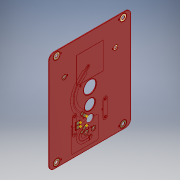
# Autodesk Inventor part: +XPanel_PCB
Saved by Autodesk Inventor 2018 (Build 220112000, 112)
## iProperties
Created: 2018-07-05
Part Number: +XPanel_PCB
Material: Epoxy Resin
Document SubType Name: Modeling
Designer: Bradley
Density: 1.14 g/cm^3
Appearance: Smooth - Red
Mass: 8.24144 g
Surface Area: 149.532 cm^2
Volume: 7.22933 cm^3
Author: Bradley
Autodesk Inventor part; units mm, degrees
(part 1 of 2)
ref_plane "YZ Plane" through (0, 0, 0) normal (1, 0, 0) x (0, 1, 0)
ref_plane "XZ Plane" through (0, 0, 0) normal (0, 1, 0) x (-1, 0, 0)
ref_plane "XY Plane" through (0, 0, 0) normal (0, 0, 1) x (1, 0, 0)
sketch "Sketch1" plane through (0, 0, 0) normal (1, 0, 0) x (0, 1, 0)
  line L0 (-35, -49.5) -> (35, -49.5)
  line L1 (40, -44.5) -> (40, 44.5)
  line L2 (35, 49.5) -> (-35, 49.5)
  line L3 (-40, 44.5) -> (-40, -44.5)
  line L4 (-40, -49.5) -> (40, 49.5) construction
  line L5 (40, -49.5) -> (-40, 49.5) construction
  arc A0 (-35, 49.5) -> (-40, 44.5) centre (-35, 44.5) ccw
  arc A1 (40, 44.5) -> (35, 49.5) centre (35, 44.5) ccw
  arc A2 (35, -49.5) -> (40, -44.5) centre (35, -44.5) ccw
  arc A3 (-40, -44.5) -> (-35, -49.5) centre (-35, -44.5) ccw
  point P0 (0, 0)
  dimension "d0" = 80
  dimension "d1" = 99
  dimension "d2" = 5
  constraints: 12 end point, 8 point on circle, 8 point on line, 8 tangent, 4 centre point, 3 equal radius, 2 midpoint, 2 parallel, 1 horizontal, 1 perpendicular
  measures "d0" distance of L4.end L5.end
  measures "d1" distance of L5.end L4.start
  measures "d2" radius of A0
extrude "Extrusion1" add sketch "Sketch1" along normal mid plane 0.5
sketch "Sketch2" plane through (0.25, 0, 0) normal (1, 0, 0) x (0, 0, -1)
  line L0 (45, -32.5) -> (-45, -32.5) construction
  line L1 (-45, -32.5) -> (-45, 32.5) construction
  line L2 (-45, 32.5) -> (45, 32.5) construction
  line L3 (45, 32.5) -> (45, -32.5) construction
  line L4 (45, -32.5) -> (-45, 32.5) construction
  line L5 (-45, -32.5) -> (45, 32.5) construction
  point P0 (0, 0)
  dimension "d5" = 90
  dimension "d6" = 65
  constraints: 12 end point, 4 coincident, 2 midpoint, 2 parallel, 1 horizontal, 1 perpendicular
  measures "d5" distance of L1.end L2.end
  measures "d6" distance of L0.end L1.end
hole "Hole1" at (0.25, -32.5, 45) at (0.25, 32.5, 45) at (0.25, 32.5, -45) at (0.25, -32.5, -45) direction (-1, 0, 0) diameter 3.3 end through all
sketch "Sketch3" plane through (0.25, 0, 0) normal (1, 0, 0) x (0, 0, -1)
  circle A0 centre (-2.5, 0) radius 6
  circle A1 centre (12.35, 0) radius 5
  circle A2 centre (-21, -1.75) radius 0.475
  circle A3 centre (24, 0) radius 3.5
  circle A4 centre (38.6, 1) radius 0.4572
  circle A5 centre (38.6, -1) radius 0.4572
  line L0 (38.6, -1) -> (38.6, 1) construction
  line L1 (38.6, 1) -> (38.6, 5.5714) construction
  line L2 (34.1, -3.5714) -> (34.1, 3.5714) construction
  line L3 (-23.3841, -25.0749) -> (-23.3841, 25.0749) construction
  line L4 (-2.5, 0) -> (-37.3972, 41.9) construction
  line L5 (-40, 41.9) -> (-5.1028, 0) construction
  line L6 (15, -15) -> (30, -15) construction
  line L7 (30, -15) -> (30, 15) construction
  line L8 (30, 15) -> (15, 15) construction
  line L9 (15, 15) -> (15, -15) construction
  circle A6 centre (15, -15) radius 0.5
  circle A7 centre (30, -15) radius 0.5
  circle A8 centre (30, 15) radius 0.5
  circle A9 centre (15, 15) radius 0.5
  circle A10 centre (0, 0) radius 39 construction
  circle A11 centre (0, 0) radius 34.2865 construction
  point P0 (38.6, 0)
  point P1 (34.1, 0)
  point P2 (30, 0)
  dimension "d53" = 78
  dimension "d14" = 14.85
  dimension "d15" = 12
  dimension "d16" = 10
  dimension "d19" = 2.5
  dimension "d20" = 21
  dimension "d21" = 1.75
  dimension "d22" = 0.95
  dimension "d23" = 7
  dimension "d24" = 26.5
  dimension "d25" = 0.9144
  dimension "d26" = 2
  dimension "d27" = 38.6
  dimension "d28" = 4.5714
  dimension "d34" = 4.5
  dimension "d46" = 2
  dimension "d47" = 41.9
  dimension "d49" = 15
  dimension "d50" = 1
  dimension "d51" = 30
  dimension "d52" = 15
  dimension "d54" = 40
  dimension "d55" = 2
  constraints: 20 end point, 11 centre point, 8 horizontal alignment, 6 coincident, 4 equal radius, 4 vertical, 3 midpoint, 3 parallel, 3 point on circle, 1 horizontal, 1 perpendicular, 1 point on line, 3 other
  measures "d14" distance of A1.centre point (-2.5, 0)
  measures "d15" diameter of A0
  measures "d16" diameter of A1
  measures "d19" distance of point (0, 0) point (-2.5, 0)
  measures "d20" horizontal distance of point (0, 0) A2.centre
  measures "d21" vertical distance of point (0, 0) A2.centre
  measures "d22" diameter of A2
  measures "d23" diameter of A3
  measures "d24" distance of A3.centre point (-2.5, 0)
  measures "d25" diameter of A4
  measures "d26" distance of L0.start L0.end
  measures "d27" distance from line of point (0, 0) L0
  measures "d28" distance of L0.end L1.end
  measures "d34" distance between parallel lines of L0 L2
  measures "d46" distance between parallel lines of L4 L5
  measures "d47" vertical distance of L4.start L4.end
  measures "d49" distance of L8.end L7.end
  measures "d50" diameter of A6
  measures "d51" distance of L6.end L7.end
  measures "d52" distance from line of point (0, 0) L9
  measures "d54" horizontal distance of point (0, 0) L5.start
  measures "d55" vertical distance of L2.end L1.end
extrude "Extrusion2" cut sketch "Sketch3" against normal through all
sketch "Sketch4" plane through (0.25, 0, 0) normal (1, 0, 0) x (0, 0, -1)
  point P0 (0, 0)
  point P1 (34.1, -3.5714)
  point P2 (34.1, 3.5714)
  point P3 (-23.3841, -25.0749)
  point P4 (-23.3841, 25.0749)
hole "Hole2" at (0.25, -3.5714, -34.1) at (0.25, 3.5714, -34.1) at (0.25, -25.0749, 23.3841) at (0.25, 25.0749, 23.3841) direction (-1, 0, 0) diameter 2.2 end through all clearance for "Flat Head Machine Screw" size "M2" standard "Ansi Metric M Profile"
sketch "Sketch5" plane through (0.25, 0, 0) normal (1, 0, 0) x (0, 0, -1)
  circle A0 centre (-23.3841, -25.0749) radius 1.1 projected
  circle A1 centre (34.1, -3.5714) radius 1.1 projected
  circle A2 centre (34.1, 3.5714) radius 1.1 projected
  circle A3 centre (-23.3841, 25.0749) radius 1.1 projected
  circle A4 centre (12.35, 0) radius 5 projected
  circle A5 centre (15, 15) radius 0.5 projected
  circle A6 centre (30, -15) radius 0.5 projected
  circle A7 centre (-21, -1.75) radius 0.475 projected
  circle A8 centre (38.6, 1) radius 0.4572 projected
  circle A9 centre (38.6, -1) radius 0.4572 projected
  circle A10 centre (15, -15) radius 0.5 projected
  circle A11 centre (30, 15) radius 0.5 projected
  circle A12 centre (24, 0) radius 3.5 projected
  circle A13 centre (-2.5, 0) radius 6 projected
  circle A14 centre (45, 32.5) radius 1.65 projected
  circle A15 centre (-45, -32.5) radius 1.65 projected
  circle A16 centre (-45, 32.5) radius 1.65 projected
  circle A17 centre (45, -32.5) radius 1.65 projected
  line L0 (-44.5, -40) -> (44.5, -40) projected
  arc A18 (44.5, -40) -> (49.5, -35) centre (44.5, -35) ccw projected
  line L1 (49.5, -35) -> (49.5, 35) projected
  arc A19 (49.5, 35) -> (44.5, 40) centre (44.5, 35) ccw projected
  line L2 (44.5, 40) -> (-44.5, 40) projected
  arc A20 (-44.5, 40) -> (-49.5, 35) centre (-44.5, 35) ccw projected
  line L3 (-49.5, 35) -> (-49.5, -35) projected
  arc A21 (-49.5, -35) -> (-44.5, -40) centre (-44.5, -35) ccw projected
  circle A22 centre (-45, -32.5) radius 1.65 projected
  circle A23 centre (-45, -32.5) radius 3
  circle A24 centre (-23.3841, -25.0749) radius 1.1 projected
  circle A25 centre (-23.3841, -25.0749) radius 2
  circle A26 centre (-45, 32.5) radius 1.65 projected
  circle A27 centre (-45, 32.5) radius 3
  circle A28 centre (-23.3841, 25.0749) radius 1.1 projected
  circle A29 centre (-23.3841, 25.0749) radius 2
  circle A30 centre (34.1, 3.5714) radius 1.1 projected
  circle A31 centre (34.1, 3.5714) radius 2
  circle A32 centre (34.1, -3.5714) radius 1.1 projected
  circle A33 centre (34.1, -3.5714) radius 2
  circle A34 centre (45, -32.5) radius 3
  circle A35 centre (45, 32.5) radius 1.65 projected
  circle A36 centre (45, 32.5) radius 3
  circle A37 centre (38.6, -1) radius 0.85
  circle A38 centre (38.6, 1) radius 0.4572 projected
  circle A39 centre (38.6, 1) radius 0.85
  circle A40 centre (30, 15) radius 0.9
  circle A41 centre (15, 15) radius 0.5 projected
  circle A42 centre (15, 15) radius 0.9
  circle A43 centre (30, -15) radius 0.5 projected
  circle A44 centre (30, -15) radius 0.9
  circle A45 centre (15, -15) radius 0.5 projected
  circle A46 centre (15, -15) radius 0.9
  line L4 (22.9, -12) -> (25.1, -12) construction
  line L5 (25.1, -12) -> (25.1, -10) construction
  line L6 (25.1, -10) -> (22.9, -10) construction
  line L7 (22.9, -10) -> (22.9, -12) construction
  line L8 (22.75, -9) -> (25.25, -9) construction
  line L9 (25.25, -9) -> (25.25, -5.5) construction
  line L10 (25.25, -5.5) -> (22.75, -5.5) construction
  line L11 (22.75, -5.5) -> (22.75, -9) construction
  line L12 (24, -10) -> (24, -9) construction
  line L13 (28.773, -3.0052) -> (27.0052, -4.773)
  line L14 (31.2478, -5.4801) -> (28.773, -3.0052)
  line L15 (27.0052, -4.773) -> (29.4801, -7.2478)
  line L16 (29.4801, -7.2478) -> (31.2478, -5.4801)
  line L17 (31.0711, -7.0711) -> (30.364, -6.364) construction
  line L18 (31.8489, -6.2933) -> (30.2933, -7.8489)
  line L19 (33.2631, -7.7075) -> (31.8489, -6.2933)
  line L20 (30.2933, -7.8489) -> (31.7075, -9.2631)
  line L21 (31.7075, -9.2631) -> (33.2631, -7.7075)
  line L22 (19.227, -3.0052) -> (16.7522, -5.4801)
  line L23 (20.9948, -4.773) -> (19.227, -3.0052)
  line L24 (18.5199, -7.2478) -> (20.9948, -4.773)
  line L25 (16.7522, -5.4801) -> (18.5199, -7.2478)
  line L26 (17.7067, -7.8489) -> (16.1511, -6.2933)
  line L27 (16.1511, -6.2933) -> (14.7369, -7.7075)
  line L28 (14.7369, -7.7075) -> (16.2925, -9.2631)
  line L29 (16.2925, -9.2631) -> (17.7067, -7.8489)
  line L30 (20.75, -13) -> (23.75, -13)
  line L31 (23.75, -13) -> (23.75, -10)
  line L32 (23.75, -10) -> (20.75, -10)
  line L33 (20.75, -10) -> (20.75, -13)
  line L34 (24.25, -13) -> (27.25, -13)
  line L35 (27.25, -13) -> (27.25, -10)
  line L36 (27.25, -10) -> (24.25, -10)
  line L37 (24.25, -10) -> (24.25, -13)
  circle A47 centre (-21, -1.75) radius 0.85
  point P0 (0, 0)
  point P1 (17.636, -6.364)
  point P2 (16.9289, -7.0711)
  dimension "d56" = 6
  dimension "d57" = 4
  dimension "d58" = 1.8
  dimension "d59" = 1.7
  dimension "d60" = 2.5
  dimension "d61" = 2.2
  dimension "d62" = 3.5
  dimension "d63" = 2
  dimension "d64" = 1
  dimension "d67" = 45
  dimension "d69" = 5.5
  dimension "d72" = 90
  dimension "d74" = 3
  dimension "d75" = 0.5
  dimension "d76" = 10
  dimension "d79" = 1.7
  constraints: 68 end point, 16 coincident, 15 centre point, 10 equal radius, 9 parallel, 6 perpendicular, 4 horizontal, 4 point on line, 2 midpoint, 40 other
  measures "d56" diameter of A23
  measures "d57" diameter of A25
  measures "d58" diameter of A46
  measures "d59" diameter of A37
  measures "d60" distance of L9.end L10.end
  measures "d61" distance of L4.start L4.end
  measures "d62" distance of L10.end L8.start
  measures "d63" distance of L6.end L4.start
  measures "d64" distance between parallel lines of L8 L6
  measures "d69" distance from line of A12.centre L10
  measures "d74" distance of L32.end L30.start
  measures "d75" distance between parallel lines of L37 L31
  measures "d76" distance from line of A12.centre L32
  measures "d79" diameter of A47
extrude "Extrusion3" add sketch "Sketch5" along normal blind 0.035 contours A23 | A25 | A27 | A29 | A31 | A33 | A34 | A36 | A37 | A39 | A40 | A42 | A44 | A46 | L14 L16 L15 L13 | L19 L21 L20 L18 | L23 L24 L25 L22 | L29 L28 L27 L26 | L33 L32 L31 L30 | L37 L36 L35 L34 | A47
sketch "Sketch6" plane through (0.25, 0, 0) normal (1, 0, 0) x (0, 0, -1)
  circle A0 centre (45, 32.5) radius 3 projected
  circle A1 centre (-45, 32.5) radius 3 projected
  circle A2 centre (34.1, -3.5714) radius 2 projected
  circle A3 centre (-23.3841, 25.0749) radius 2 projected
  line L0 (24.25, -13) -> (24.25, -10) projected
  line L1 (24.25, -10) -> (27.25, -10) projected
  line L2 (27.25, -10) -> (27.25, -13) projected
  line L3 (27.25, -13) -> (24.25, -13) projected
  line L4 (20.9948, -4.773) -> (18.5199, -7.2478) projected
  line L5 (18.5199, -7.2478) -> (16.7522, -5.4801) projected
  line L6 (16.7522, -5.4801) -> (19.227, -3.0052) projected
  line L7 (19.227, -3.0052) -> (20.9948, -4.773) projected
  line L8 (16.2925, -9.2631) -> (14.7369, -7.7075) projected
  line L9 (14.7369, -7.7075) -> (16.1511, -6.2933) projected
  line L10 (16.1511, -6.2933) -> (17.7067, -7.8489) projected
  line L11 (17.7067, -7.8489) -> (16.2925, -9.2631) projected
  circle A4 centre (-21, -1.75) radius 0.85 projected
  circle A5 centre (30, -15) radius 0.9 projected
  circle A6 centre (30, 15) radius 0.9 projected
  circle A7 centre (38.6, -1) radius 0.85 projected
  circle A8 centre (38.6, 1) radius 0.85 projected
  circle A9 centre (15, 15) radius 0.9 projected
  circle A10 centre (15, -15) radius 0.9 projected
  line L12 (33.2631, -7.7075) -> (31.7075, -9.2631) projected
  line L13 (31.7075, -9.2631) -> (30.2933, -7.8489) projected
  line L14 (30.2933, -7.8489) -> (31.8489, -6.2933) projected
  line L15 (31.8489, -6.2933) -> (33.2631, -7.7075) projected
  line L16 (31.2478, -5.4801) -> (29.4801, -7.2478) projected
  line L17 (29.4801, -7.2478) -> (27.0052, -4.773) projected
  line L18 (27.0052, -4.773) -> (28.773, -3.0052) projected
  line L19 (28.773, -3.0052) -> (31.2478, -5.4801) projected
  line L20 (20.75, -13) -> (20.75, -10) projected
  line L21 (20.75, -10) -> (23.75, -10) projected
  line L22 (23.75, -10) -> (23.75, -13) projected
  line L23 (23.75, -13) -> (20.75, -13) projected
  circle A11 centre (-23.3841, -25.0749) radius 2 projected
  circle A12 centre (34.1, 3.5714) radius 2 projected
  circle A13 centre (-45, -32.5) radius 3 projected
  circle A14 centre (45, -32.5) radius 3 projected
  circle A15 centre (12.35, 0) radius 5 projected
  circle A16 centre (24, 0) radius 3.5 projected
  circle A17 centre (-2.5, 0) radius 6 projected
  line L24 (-44.5, -40) -> (44.5, -40) projected
  arc A18 (44.5, -40) -> (49.5, -35) centre (44.5, -35) ccw projected
  line L25 (49.5, -35) -> (49.5, 35) projected
  arc A19 (49.5, 35) -> (44.5, 40) centre (44.5, 35) ccw projected
  line L26 (44.5, 40) -> (-44.5, 40) projected
  arc A20 (-44.5, 40) -> (-49.5, 35) centre (-44.5, 35) ccw projected
  line L27 (-49.5, 35) -> (-49.5, -35) projected
  arc A21 (-49.5, -35) -> (-44.5, -40) centre (-44.5, -35) ccw projected
  line L28 (-21, -1.75) -> (-12.1029, -10.6471) construction
  arc A22 (-12.1029, -10.6471) -> (13.3529, -10.6471) centre (0.625, 2.0808) ccw construction
  line L29 (13.3529, -10.6471) -> (15.5147, -8.4853) construction
  line L30 (14.7369, -7.7075) -> (16.2925, -9.2631) projected
  line L31 (16.1511, -6.2933) -> (14.7369, -7.7075) projected
  line L32 (33.2631, -7.7075) -> (31.7075, -9.2631) projected
  arc A23 (32.4853, -8.4853) -> (38.6, -5.9525) centre (35.0181, -5.9525) ccw construction
  line L33 (31.7075, -9.2631) -> (33.2631, -7.7075) projected
  circle A24 centre (38.6, -1) radius 0.85 construction
  line L34 (38.6, -1) -> (38.6, -5.9525) construction
  arc A25 (33.2631, -7.7075) -> (37.5, -5.9525) centre (35.0181, -5.9525) ccw
  line L35 (37.5, -5.9525) -> (37.5, -1.5123)
  arc A26 (31.7075, -9.2631) -> (39.7, -5.9525) centre (35.0181, -5.9525) ccw
  line L36 (39.7, -5.9525) -> (39.7, -1.5123)
  line L37 (31.7075, -9.2631) -> (33.2631, -7.7075)
  line L38 (15.1612, -8.1317) -> (12.9994, -10.2935)
  arc A27 (-11.7494, -10.2935) -> (12.9994, -10.2935) centre (0.625, 2.0808) ccw
  line L39 (-11.7494, -10.2935) -> (-20.1604, -1.8825)
  line L40 (15.8683, -8.8388) -> (13.7065, -11.0006)
  arc A28 (-12.4565, -11.0006) -> (13.7065, -11.0006) centre (0.625, 2.0808) ccw
  line L41 (-12.4565, -11.0006) -> (-20.8675, -2.5896)
  circle A29 centre (-21, -1.75) radius 0.85 projected
  arc A30 (30.7882, -10.1823) -> (41, -5.9525) centre (35.0181, -5.9525) ccw construction
  line L42 (41, -5.9525) -> (41, -0.6805) construction
  arc A31 (39.7, -1.5123) -> (39.1231, -0.33) centre (38.2, -1.5123) ccw
  arc A32 (38.0769, -0.33) -> (37.5, -1.5123) centre (39, -1.5123) ccw
  arc A33 (41, -0.6805) -> (38.6, 1) centre (39.2117, -0.6805) ccw construction
  line L43 (30.7882, -10.1823) -> (29.374, -8.7681) construction
  arc A34 (28.9347, -7.7075) -> (29.374, -8.7681) centre (30.4347, -7.7075) ccw construction
  arc A35 (30.0347, -7.7075) -> (30.1518, -7.9903) centre (30.4347, -7.7075) ccw
  line L44 (30.1518, -7.9903) -> (31.566, -9.4045)
  arc A36 (31.566, -9.4045) -> (39.9, -5.9525) centre (35.0181, -5.9525) ccw
  line L45 (39.9, -5.9525) -> (39.9, -0.6805)
  arc A37 (39.9, -0.6805) -> (39.1502, 0.0051) centre (39.2117, -0.6805) ccw
  arc A38 (27.8347, -7.7075) -> (28.5962, -9.5459) centre (30.4347, -7.7075) ccw
  line L46 (28.5962, -9.5459) -> (30.0104, -10.9602)
  arc A39 (30.0104, -10.9602) -> (42.1, -5.9525) centre (35.0181, -5.9525) ccw
  line L47 (42.1, -5.9525) -> (42.1, -0.6805)
  arc A40 (42.1, -0.6805) -> (39.1468, 2.2071) centre (39.2117, -0.6805) ccw
  line L48 (30.2933, -7.8489) -> (31.7075, -9.2631) projected
  circle A41 centre (38.6, 1) radius 0.85 projected
  arc A42 (38.0555, 0.3473) -> (39.1502, 0.0051) centre (39.0164, 1.4991) ccw
  arc A43 (39.1468, 2.2071) -> (37.8409, 1.3825) centre (39.1805, 0.7075) ccw
  circle A44 centre (38.6, 1) radius 0.85 projected
  line L49 (31.8489, -6.2933) -> (30.2933, -7.8489) projected
  line L50 (30.0347, -7.7075) -> (30.0347, -6.6933)
  line L51 (27.8347, -7.7075) -> (27.8347, -5.6024)
  line L52 (28.9347, -7.7075) -> (28.9347, -6.7024) construction
  line L53 (-49.2, -35) -> (-49.2, 35)
  arc A45 (-44.5, 39.7) -> (-49.2, 35) centre (-44.5, 35) ccw
  line L54 (-44.5, 39.7) -> (44.5, 39.7)
  arc A46 (49.2, 35) -> (44.5, 39.7) centre (44.5, 35) ccw
  line L55 (49.2, 35) -> (49.2, -35)
  arc A47 (44.5, -39.7) -> (49.2, -35) centre (44.5, -35) ccw
  line L56 (44.5, -39.7) -> (-44.5, -39.7)
  arc A48 (-49.2, -35) -> (-44.5, -39.7) centre (-44.5, -35) ccw
  circle A49 centre (-45, -32.5) radius 3.3
  circle A50 centre (-45, 32.5) radius 3.3
  circle A51 centre (-23.3841, 25.0749) radius 2.3
  circle A52 centre (-23.3841, -25.0749) radius 2.3
  circle A53 centre (-2.5, 0) radius 6.3
  circle A54 centre (12.35, 0) radius 5.3
  circle A55 centre (45, 32.5) radius 3.3
  circle A56 centre (45, -32.5) radius 3.3
  arc A57 (-19.9393, -0.6893) -> (-22.0607, -2.8107) centre (-21, -1.75) ccw
  line L57 (-19.9393, -0.6893) -> (-17.7751, -2.8536)
  arc A58 (-17.7751, -2.8536) -> (-17.4216, -3) centre (-17.4216, -2.5) ccw
  line L58 (-17.4216, -3) -> (-15.7145, -3)
  arc A59 (-15.3609, -3.1464) -> (-15.7145, -3) centre (-15.7145, -3.5) ccw
  line L59 (-15.3609, -3.1464) -> (-9.9816, -8.5258)
  arc A60 (-9.9816, -8.5258) -> (11.2316, -8.5258) centre (0.625, 2.0808) ccw
  line L60 (11.2316, -8.5258) -> (14.1308, -5.6265)
  line L61 (-22.0607, -2.8107) -> (-19.8964, -4.9749)
  arc A61 (-19.75, -5.3284) -> (-19.8964, -4.9749) centre (-20.25, -5.3284) ccw
  line L62 (-19.75, -5.3284) -> (-19.75, -7.0355)
  arc A62 (-19.75, -7.0355) -> (-19.6036, -7.3891) centre (-19.25, -7.0355) ccw
  line L63 (-19.6036, -7.3891) -> (-14.2242, -12.7684)
  arc A63 (-14.2242, -12.7684) -> (15.4742, -12.7684) centre (0.625, 2.0808) ccw
  line L64 (15.4742, -12.7684) -> (18.3735, -9.8692)
  arc A64 (14.4844, -5.4801) -> (14.1308, -5.6265) centre (14.4844, -5.9801) ccw
  line L65 (14.4844, -5.4801) -> (16.7522, -5.4801)
  arc A65 (18.3735, -9.8692) -> (18.5199, -9.5156) centre (18.0199, -9.5156) ccw
  line L66 (18.5199, -9.5156) -> (18.5199, -7.2478)
  circle A66 centre (21.25, -13.5) radius 0.225
  circle A67 centre (24.75, -13.5) radius 0.225
  circle A68 centre (22.25, -13.5) radius 0.225
  circle A69 centre (25.75, -13.5) radius 0.225
  circle A70 centre (23.25, -13.5) radius 0.225
  circle A71 centre (26.75, -13.5) radius 0.225
  line L67 (24.25, -13) -> (27.25, -13) projected
  line L68 (24.25, -13) -> (24.25, -13.5)
  arc A72 (24.25, -13.5) -> (24.75, -14) centre (24.75, -13.5) ccw
  line L69 (24.75, -14) -> (26.75, -14)
  arc A73 (26.75, -14) -> (27.25, -13.5) centre (26.75, -13.5) ccw
  line L70 (27.25, -10) -> (27.25, -13) projected
  line L71 (27.25, -13.5) -> (27.25, -13)
  line L72 (23.75, -13) -> (23.75, -13.5)
  arc A74 (23.25, -14) -> (23.75, -13.5) centre (23.25, -13.5) ccw
  line L73 (23.25, -14) -> (21.25, -14)
  arc A75 (20.75, -13.5) -> (21.25, -14) centre (21.25, -13.5) ccw
  line L74 (20.75, -13.5) -> (20.75, -13)
  circle A76 centre (15, -15) radius 0.9 projected
  circle A77 centre (15, -15) radius 1.2
  circle A78 centre (30, -15) radius 0.9 projected
  circle A79 centre (30, 15) radius 1.2
  circle A80 centre (15, 15) radius 1.2
  line L75 (20.45, -10) -> (20.45, -13.5)
  arc A81 (20.45, -13.5) -> (21.25, -14.3) centre (21.25, -13.5) ccw
  arc A82 (20.75, -9.7) -> (20.45, -10) centre (20.75, -10) ccw
  line L76 (21.25, -14.3) -> (24, -14.3)
  line L77 (24, -14.3) -> (24, -17)
  arc A83 (24, -17) -> (25, -18) centre (25, -17) ccw
  line L78 (25, -18) -> (45, -18)
  arc A84 (45, -18) -> (46, -17) centre (45, -17) ccw
  line L79 (46, -17) -> (46, 7)
  arc A85 (46, 7) -> (45, 8) centre (45, 7) ccw
  line L80 (45, 8) -> (25, 8)
  arc A86 (25, 8) -> (24, 7) centre (25, 7) ccw
  line L81 (24, 7) -> (24, 3.8)
  arc A87 (24, 3.8) -> (24, -3.8) centre (24, 0) ccw
  line L82 (20.75, -9.7) -> (24, -9.7)
  line L83 (24, -9.7) -> (24, -3.8)
  arc A88 (39.1231, -0.33) -> (38.0769, -0.33) centre (38.6, -1) ccw
  point P0 (0, 0)
  point P1 (25.75, -13)
  dimension "d80" = 18
  dimension "d81" = 2.2
  dimension "d82" = 1
  dimension "d83" = 1.5
  dimension "d84" = 2.2
  dimension "d85" = 0.2
  dimension "d86" = 110
  dimension "d87" = 1.5
  dimension "d88" = 0.3
  dimension "d89" = 0.3
  dimension "d90" = 0.3
  dimension "d91" = 0.3
  dimension "d92" = 0.3
  dimension "d93" = 1.5
  dimension "d94" = 3
  dimension "d95" = 0.5
  dimension "d96" = 3
  dimension "d97" = 0.45
  dimension "d100" = 1
  dimension "d105" = 1
  dimension "d106" = 0.3
  dimension "d107" = 0.3
  dimension "d108" = 0.3
  dimension "d110" = 18
  dimension "d111" = 1
  dimension "d112" = 22
  dimension "d113" = 8
  constraints: 97 end point, 94 point on circle, 61 centre point, 54 tangent, 18 equal radius, 14 perpendicular, 9 parallel, 8 concentric, 8 point on line, 7 vertical, 6 coincident, 5 collinear, 5 horizontal, 3 midpoint, 2 equal length, 1 line through centre, 1 vertical alignment, 34 other
  measures "d80" radius of A22
  measures "d81" distance between parallel lines of L36 L35
  measures "d82" distance between parallel lines of L39 L41
  measures "d83" radius of A32
  measures "d84" distance between parallel lines of L47 L45
  measures "d85" distance between parallel lines of L45 L36
  measures "d87" radius of A34
  measures "d88" distance between parallel lines of L27 L53
  measures "d89" radial gap between concentric circles of A13 A49
  measures "d90" radial gap between concentric circles of A11 A52
  measures "d91" radial gap between concentric circles of A17 A53
  measures "d92" radial gap between concentric circles of A54 A15
  measures "d93" radius of A57
  measures "d94" distance between parallel lines of L59 L28
  measures "d95" radius of A58
  measures "d96" distance from line of point (0, 0) L58
  measures "d97" diameter of A66
  measures "d100" distance of A66.centre A68.centre
  measures "d105" distance between parallel lines of L23 L73
  measures "d106" radial gap between concentric circles of A77 A10
  measures "d107" distance between parallel lines of L75 L74
  measures "d108" radial gap between concentric circles of A16 A87
  measures "d110" distance from line of A87.centre L78
  measures "d111" radius of A83
  measures "d112" distance from line of L79 A16.centre
  measures "d113" distance from line of L80 A16.centre
extrude "Extrusion4" add sketch "Sketch6" along normal blind 0.05 contours L3 L71 A73 L69 A72 L68 | L40 A28 L41 A4 L39 A27 L38 L8 | A7 A31 L36 A26 L12 A25 L35 A32 | A8 A43 A40 L47 A39 L46 A38 L51 L17 L16 L50 A35 L44 A36 L45 A37 A42 | L23 L72 A74 L73 A75 L74 | L53 A45 L54 A46 L55 A47 L56 A48
sketch "Sketch7" plane through (0.25, 0, 0) normal (1, 0, 0) x (0, 0, -1)
  circle A0 centre (24, 0) radius 3.5 projected
  circle A1 centre (34.1, 3.5714) radius 2 projected
  circle A2 centre (30, -15) radius 0.9 projected
  circle A3 centre (34.1, -3.5714) radius 2 projected
  arc A4 (20.75, -9.7) -> (20.45, -10) centre (20.75, -10) ccw projected
  line L0 (20.45, -10) -> (20.45, -13.5) projected
  arc A5 (20.45, -13.5) -> (21.25, -14.3) centre (21.25, -13.5) ccw projected
  line L1 (21.25, -14.3) -> (24, -14.3) projected
  line L2 (24, -14.3) -> (24, -17) projected
  arc A6 (24, -17) -> (25, -18) centre (25, -17) ccw projected
  line L3 (25, -18) -> (45, -18) projected
  arc A7 (45, -18) -> (46, -17) centre (45, -17) ccw projected
  line L4 (46, -17) -> (46, 7) projected
  arc A8 (46, 7) -> (45, 8) centre (45, 7) ccw projected
  line L5 (45, 8) -> (25, 8) projected
  arc A9 (25, 8) -> (24, 7) centre (25, 7) ccw projected
  line L6 (24, 7) -> (24, 3.8) projected
  arc A10 (24, 3.8) -> (24, -3.8) centre (24, 0) ccw projected
  line L7 (24, -3.8) -> (24, -9.7) projected
  line L8 (24, -9.7) -> (20.75, -9.7) projected
  arc A11 (38.0769, -0.33) -> (37.5, -1.5123) centre (39, -1.5123) ccw projected
  arc A12 (39.1231, -0.33) -> (38.0769, -0.33) centre (38.6, -1) ccw projected
  arc A13 (39.7, -1.5123) -> (39.1231, -0.33) centre (38.2, -1.5123) ccw projected
  line L9 (39.7, -1.5123) -> (39.7, -5.9525) projected
  arc A14 (31.7075, -9.2631) -> (39.7, -5.9525) centre (35.0181, -5.9525) ccw projected
  line L10 (31.7075, -9.2631) -> (30.2933, -7.8489) projected
  line L11 (30.2933, -7.8489) -> (31.8489, -6.2933) projected
  line L12 (31.8489, -6.2933) -> (33.2631, -7.7075) projected
  arc A15 (33.2631, -7.7075) -> (37.5, -5.9525) centre (35.0181, -5.9525) ccw projected
  line L13 (37.5, -5.9525) -> (37.5, -1.5123) projected
  line L14 (24.25, -13.5) -> (24.25, -10) projected
  line L15 (24.25, -10) -> (27.25, -10) projected
  line L16 (27.25, -10) -> (27.25, -13.5) projected
  arc A16 (26.75, -14) -> (27.25, -13.5) centre (26.75, -13.5) ccw projected
  line L17 (26.75, -14) -> (24.75, -14) projected
  arc A17 (24.25, -13.5) -> (24.75, -14) centre (24.75, -13.5) ccw projected
  line L18 (20.75, -13.5) -> (20.75, -10) projected
  line L19 (20.75, -10) -> (23.75, -10) projected
  line L20 (23.75, -10) -> (23.75, -13.5) projected
  arc A18 (23.25, -14) -> (23.75, -13.5) centre (23.25, -13.5) ccw projected
  line L21 (23.25, -14) -> (21.25, -14) projected
  arc A19 (20.75, -13.5) -> (21.25, -14) centre (21.25, -13.5) ccw projected
  arc A20 (38.0555, 0.3473) -> (39.1502, 0.0051) centre (39.0164, 1.4991) ccw projected
  arc A21 (37.8409, 1.3825) -> (38.0555, 0.3473) centre (38.6, 1) ccw projected
  arc A22 (39.1468, 2.2071) -> (37.8409, 1.3825) centre (39.1805, 0.7075) ccw projected
  arc A23 (42.1, -0.6805) -> (39.1468, 2.2071) centre (39.2117, -0.6805) ccw projected
  line L22 (42.1, -0.6805) -> (42.1, -5.9525) projected
  arc A24 (30.0104, -10.9602) -> (42.1, -5.9525) centre (35.0181, -5.9525) ccw projected
  line L23 (30.0104, -10.9602) -> (28.5962, -9.5459) projected
  arc A25 (27.8347, -7.7075) -> (28.5962, -9.5459) centre (30.4347, -7.7075) ccw projected
  line L24 (27.8347, -7.7075) -> (27.8347, -5.6024) projected
  line L25 (27.8347, -5.6024) -> (27.0052, -4.773) projected
  line L26 (27.0052, -4.773) -> (28.773, -3.0052) projected
  line L27 (28.773, -3.0052) -> (31.2478, -5.4801) projected
  line L28 (31.2478, -5.4801) -> (30.0347, -6.6933) projected
  line L29 (30.0347, -6.6933) -> (30.0347, -7.7075) projected
  arc A26 (30.0347, -7.7075) -> (30.1518, -7.9903) centre (30.4347, -7.7075) ccw projected
  line L30 (30.1518, -7.9903) -> (31.566, -9.4045) projected
  arc A27 (31.566, -9.4045) -> (39.9, -5.9525) centre (35.0181, -5.9525) ccw projected
  line L31 (39.9, -5.9525) -> (39.9, -0.6805) projected
  arc A28 (39.9, -0.6805) -> (39.1502, 0.0051) centre (39.2117, -0.6805) ccw projected
  line L32 (12.9994, -10.2935) -> (15.1612, -8.1317) projected
  line L33 (15.1612, -8.1317) -> (14.7369, -7.7075) projected
  line L34 (14.7369, -7.7075) -> (16.1511, -6.2933) projected
  line L35 (16.1511, -6.2933) -> (17.7067, -7.8489) projected
  line L36 (17.7067, -7.8489) -> (16.2925, -9.2631) projected
  line L37 (16.2925, -9.2631) -> (15.8683, -8.8388) projected
  line L38 (15.8683, -8.8388) -> (13.7065, -11.0006) projected
  arc A29 (-12.4565, -11.0006) -> (13.7065, -11.0006) centre (0.625, 2.0808) ccw projected
  line L39 (-12.4565, -11.0006) -> (-20.8675, -2.5896) projected
  arc A30 (-20.1604, -1.8825) -> (-20.8675, -2.5896) centre (-21, -1.75) ccw projected
  line L40 (-20.1604, -1.8825) -> (-11.7494, -10.2935) projected
  arc A31 (-11.7494, -10.2935) -> (12.9994, -10.2935) centre (0.625, 2.0808) ccw projected
  line L41 (18.5199, -9.5156) -> (18.5199, -7.2478) projected
  line L42 (18.5199, -7.2478) -> (16.7522, -5.4801) projected
  line L43 (16.7522, -5.4801) -> (14.4844, -5.4801) projected
  arc A32 (14.4844, -5.4801) -> (14.1308, -5.6265) centre (14.4844, -5.9801) ccw projected
  line L44 (14.1308, -5.6265) -> (11.2316, -8.5258) projected
  arc A33 (-9.9816, -8.5258) -> (11.2316, -8.5258) centre (0.625, 2.0808) ccw projected
  line L45 (-9.9816, -8.5258) -> (-15.3609, -3.1464) projected
  arc A34 (-15.3609, -3.1464) -> (-15.7145, -3) centre (-15.7145, -3.5) ccw projected
  line L46 (-15.7145, -3) -> (-17.4216, -3) projected
  arc A35 (-17.7751, -2.8536) -> (-17.4216, -3) centre (-17.4216, -2.5) ccw projected
  line L47 (-17.7751, -2.8536) -> (-19.9393, -0.6893) projected
  arc A36 (-19.9393, -0.6893) -> (-22.0607, -2.8107) centre (-21, -1.75) ccw projected
  line L48 (-22.0607, -2.8107) -> (-19.8964, -4.9749) projected
  arc A37 (-19.75, -5.3284) -> (-19.8964, -4.9749) centre (-20.25, -5.3284) ccw projected
  line L49 (-19.75, -5.3284) -> (-19.75, -7.0355) projected
  arc A38 (-19.75, -7.0355) -> (-19.6036, -7.3891) centre (-19.25, -7.0355) ccw projected
  line L50 (-19.6036, -7.3891) -> (-14.2242, -12.7684) projected
  arc A39 (-14.2242, -12.7684) -> (15.4742, -12.7684) centre (0.625, 2.0808) ccw projected
  line L51 (15.4742, -12.7684) -> (18.3735, -9.8692) projected
  arc A40 (18.3735, -9.8692) -> (18.5199, -9.5156) centre (18.0199, -9.5156) ccw projected
  arc A41 (20.75, -9.7) -> (20.45, -10) centre (20.75, -10) ccw projected
  line L52 (20.75, -9.7) -> (24, -9.7) projected
  line L53 (24, -9.7) -> (24, -3.8) projected
  arc A42 (24, 3.8) -> (24, -3.8) centre (24, 0) ccw projected
  line L54 (24, 3.8) -> (24, 7) projected
  arc A43 (25, 8) -> (24, 7) centre (25, 7) ccw projected
  line L55 (25, 8) -> (45, 8) projected
  arc A44 (46, 7) -> (45, 8) centre (45, 7) ccw projected
  line L56 (46, 7) -> (46, -17) projected
  arc A45 (45, -18) -> (46, -17) centre (45, -17) ccw projected
  line L57 (45, -18) -> (25, -18) projected
  arc A46 (24, -17) -> (25, -18) centre (25, -17) ccw projected
  line L58 (24, -17) -> (24, -14.3) projected
  line L59 (24, -14.3) -> (21.25, -14.3) projected
  arc A47 (20.45, -13.5) -> (21.25, -14.3) centre (21.25, -13.5) ccw projected
  line L60 (20.45, -13.5) -> (20.45, -10) projected
  line L61 (-49.2, 35) -> (-49.2, -35) projected
  arc A48 (-49.2, -35) -> (-44.5, -39.7) centre (-44.5, -35) ccw projected
  line L62 (-44.5, -39.7) -> (44.5, -39.7) projected
  arc A49 (44.5, -39.7) -> (49.2, -35) centre (44.5, -35) ccw projected
  line L63 (49.2, -35) -> (49.2, 35) projected
  arc A50 (49.2, 35) -> (44.5, 39.7) centre (44.5, 35) ccw projected
  line L64 (44.5, 39.7) -> (-44.5, 39.7) projected
  arc A51 (-44.5, 39.7) -> (-49.2, 35) centre (-44.5, 35) ccw projected
  circle A52 centre (15, -15) radius 1.2 projected
  circle A53 centre (30, 15) radius 1.2 projected
  circle A54 centre (15, 15) radius 1.2 projected
  line L65 (18.5199, -7.2478) -> (18.5199, -9.5156) projected
  arc A55 (18.3735, -9.8692) -> (18.5199, -9.5156) centre (18.0199, -9.5156) ccw projected
  line L66 (18.3735, -9.8692) -> (15.4742, -12.7684) projected
  arc A56 (-14.2242, -12.7684) -> (15.4742, -12.7684) centre (0.625, 2.0808) ccw projected
  line L67 (-14.2242, -12.7684) -> (-19.6036, -7.3891) projected
  arc A57 (-19.75, -7.0355) -> (-19.6036, -7.3891) centre (-19.25, -7.0355) ccw projected
  line L68 (-19.75, -7.0355) -> (-19.75, -5.3284) projected
  arc A58 (-19.75, -5.3284) -> (-19.8964, -4.9749) centre (-20.25, -5.3284) ccw projected
  line L69 (-19.8964, -4.9749) -> (-22.0607, -2.8107) projected
  arc A59 (-19.9393, -0.6893) -> (-22.0607, -2.8107) centre (-21, -1.75) ccw projected
  line L70 (-19.9393, -0.6893) -> (-17.7751, -2.8536) projected
  arc A60 (-17.7751, -2.8536) -> (-17.4216, -3) centre (-17.4216, -2.5) ccw projected
  line L71 (-17.4216, -3) -> (-15.7145, -3) projected
  arc A61 (-15.3609, -3.1464) -> (-15.7145, -3) centre (-15.7145, -3.5) ccw projected
  line L72 (-15.3609, -3.1464) -> (-9.9816, -8.5258) projected
  arc A62 (-9.9816, -8.5258) -> (11.2316, -8.5258) centre (0.625, 2.0808) ccw projected
  line L73 (11.2316, -8.5258) -> (14.1308, -5.6265) projected
  arc A63 (14.4844, -5.4801) -> (14.1308, -5.6265) centre (14.4844, -5.9801) ccw projected
  line L74 (14.4844, -5.4801) -> (16.7522, -5.4801) projected
  line L75 (16.7522, -5.4801) -> (19.227, -3.0052) projected
  line L76 (19.227, -3.0052) -> (20.9948, -4.773) projected
  line L77 (20.9948, -4.773) -> (18.5199, -7.2478) projected
  circle A64 centre (-23.3841, 25.0749) radius 2.3 projected
  circle A65 centre (-23.3841, -25.0749) radius 2.3 projected
  circle A66 centre (-45, -32.5) radius 3.3 projected
  circle A67 centre (-45, 32.5) radius 3.3 projected
  circle A68 centre (45, 32.5) radius 3.3 projected
  circle A69 centre (45, -32.5) radius 3.3 projected
  circle A70 centre (12.35, 0) radius 5.3 projected
  circle A71 centre (-2.5, 0) radius 6.3 projected
  circle A72 centre (-45, -32.5) radius 3.5 construction
  circle A73 centre (-45, -32.5) radius 3.425
  circle A74 centre (-45, -32.5) radius 3.575
  circle A75 centre (-45, 32.5) radius 3.425
  circle A76 centre (-45, 32.5) radius 3.575
  circle A77 centre (-23.3841, 25.0749) radius 1.1 projected
  circle A78 centre (-23.3841, 25.0749) radius 2.325
  circle A79 centre (-23.3841, 25.0749) radius 2.175
  circle A80 centre (-23.3841, -25.0749) radius 2.325
  circle A81 centre (-23.3841, -25.0749) radius 2.175
  circle A82 centre (-2.5, 0) radius 6.575
  circle A83 centre (-2.5, 0) radius 6.425
  circle A84 centre (45, -32.5) radius 1.65 projected
  circle A85 centre (45, -32.5) radius 3.575
  circle A86 centre (45, -32.5) radius 3.425
  circle A87 centre (45, 32.5) radius 1.65 projected
  circle A88 centre (45, 32.5) radius 3.575
  circle A89 centre (45, 32.5) radius 3.425
  circle A90 centre (34.1, -3.5714) radius 1.1 projected
  circle A91 centre (34.1, -3.5714) radius 2.175
  circle A92 centre (34.1, -3.5714) radius 2.325
  circle A93 centre (34.1, 3.5714) radius 2.175
  circle A94 centre (34.1, 3.5714) radius 2.325
  circle A95 centre (12.35, 0) radius 5.425
  circle A96 centre (12.35, 0) radius 5.575
  circle A97 centre (-23.3841, -25.0749) radius 1.1 construction
  circle A98 centre (-23.3841, -25.0749) radius 2.25 construction
  circle A99 centre (-2.5, 0) radius 6.5 construction
  circle A100 centre (12.35, 0) radius 5.5 construction
  line L78 (-35.75, -13) -> (-9.75, -13) construction
  line L79 (-9.75, -13) -> (-9.75, 13) construction
  line L80 (-9.75, 13) -> (-35.75, 13) construction
  line L81 (-35.75, 13) -> (-35.75, -13) construction
  line L82 (-35.825, -13.075) -> (-9.675, -13.075)
  line L83 (-9.675, -13.075) -> (-9.675, 13.075)
  line L84 (-9.675, 13.075) -> (-35.825, 13.075)
  line L85 (-35.825, 13.075) -> (-35.825, -13.075)
  line L86 (-35.675, -12.925) -> (-9.825, -12.925)
  line L87 (-9.825, -12.925) -> (-9.825, 12.925)
  line L88 (-9.825, 12.925) -> (-35.675, 12.925)
  line L89 (-35.675, 12.925) -> (-35.675, -12.925)
  circle A101 centre (15, 15) radius 0.5 projected
  line L90 (15, 15) -> (30, 15) construction
  line L91 (15, 17.25) -> (30, 17.25) construction
  line L92 (30, 12.75) -> (15, 12.75) construction
  arc A102 (15, 17.25) -> (15, 12.75) centre (15, 15) ccw construction
  arc A103 (30, 12.75) -> (30, 17.25) centre (30, 15) ccw construction
  circle A104 centre (15, -15) radius 0.5 construction
  line L93 (15, -15) -> (30, -15) construction
  line L94 (15, -12.75) -> (30, -12.75) construction
  line L95 (30, -17.25) -> (15, -17.25) construction
  arc A105 (15, -12.75) -> (15, -17.25) centre (15, -15) ccw construction
  arc A106 (30, -17.25) -> (30, -12.75) centre (30, -15) ccw construction
  line L96 (15, 12.675) -> (30, 12.675)
  arc A107 (30, 12.675) -> (30, 17.325) centre (30, 15) ccw
  line L97 (30, 17.325) -> (15, 17.325)
  arc A108 (15, 17.325) -> (15, 12.675) centre (15, 15) ccw
  line L98 (15, 12.825) -> (30, 12.825)
  arc A109 (30, 12.825) -> (30, 17.175) centre (30, 15) ccw
  line L99 (30, 17.175) -> (15, 17.175)
  arc A110 (15, 17.175) -> (15, 12.825) centre (15, 15) ccw
  line L100 (15, -17.325) -> (30, -17.325)
  arc A111 (30, -17.325) -> (30, -12.675) centre (30, -15) ccw
  line L101 (30, -12.675) -> (15, -12.675)
  arc A112 (15, -12.675) -> (15, -17.325) centre (15, -15) ccw
  line L102 (15, -17.175) -> (30, -17.175)
  arc A113 (30, -17.175) -> (30, -12.825) centre (30, -15) ccw
  line L103 (30, -12.825) -> (15, -12.825)
  arc A114 (15, -12.825) -> (15, -17.175) centre (15, -15) ccw
  line L104 (20.55, -12.825) -> (20.55, -12.675)
  line L105 (27.45, -12.825) -> (27.45, -12.675)
  line L106 (14.2773, -7.6014) -> (19.227, -2.6517) construction
  line L107 (19.227, -2.6517) -> (21.3483, -4.773) construction
  line L108 (21.3483, -4.773) -> (16.3986, -9.7227) construction
  line L109 (16.3986, -9.7227) -> (14.2773, -7.6014) construction
  line L110 (14.1712, -7.6014) -> (19.227, -2.5456)
  line L111 (19.227, -2.5456) -> (21.4544, -4.773)
  line L112 (21.4544, -4.773) -> (16.3986, -9.8288)
  line L113 (16.3986, -9.8288) -> (14.1712, -7.6014)
  line L114 (14.3833, -7.6014) -> (19.227, -2.7577)
  line L115 (19.227, -2.7577) -> (21.2423, -4.773)
  line L116 (21.2423, -4.773) -> (16.3986, -9.6167)
  line L117 (16.3986, -9.6167) -> (14.3833, -7.6014)
  line L118 (33.8288, -7.6014) -> (31.6014, -9.8288)
  line L119 (33.6167, -7.6014) -> (31.6014, -9.6167)
  line L120 (31.6014, -9.8288) -> (26.5456, -4.773)
  line L121 (31.6014, -9.6167) -> (26.7577, -4.773)
  line L122 (28.773, -2.7577) -> (33.6167, -7.6014)
  line L123 (28.773, -2.5456) -> (33.8288, -7.6014)
  line L124 (26.5456, -4.773) -> (28.773, -2.5456)
  line L125 (26.7577, -4.773) -> (28.773, -2.7577)
  line L126 (20.5, -14.25) -> (27.5, -14.25) construction
  line L127 (27.5, -14.25) -> (27.5, -9.75) construction
  line L128 (27.5, -9.75) -> (20.5, -9.75) construction
  line L129 (20.5, -9.75) -> (20.5, -14.25) construction
  line L130 (20.425, -14.325) -> (27.575, -14.325)
  line L131 (27.575, -14.325) -> (27.575, -9.675)
  line L132 (27.575, -9.675) -> (20.425, -9.675)
  line L133 (20.425, -9.675) -> (20.425, -14.325)
  line L134 (20.575, -14.175) -> (27.425, -14.175)
  line L135 (27.425, -14.175) -> (27.425, -9.825)
  line L136 (27.425, -9.825) -> (20.575, -9.825)
  line L137 (20.575, -9.825) -> (20.575, -14.175)
  line L138 (-8.7724, -8.558) -> (-6.6415, -8.558) construction
  line L139 (-6.6415, -8.558) -> (-6.6415, -9.36) construction
  line L140 (-6.6415, -9.36) -> (-8.7724, -9.36) construction
  line L141 (-8.7724, -9.36) -> (-8.7724, -8.558) construction
  line L142 (40.1829, 0.0151) -> (42.3139, 0.0151) construction
  line L143 (42.3139, 0.0151) -> (42.3139, -0.7869) construction
  line L144 (42.3139, -0.7869) -> (40.1829, -0.7869) construction
  line L145 (40.1829, -0.7869) -> (40.1829, 0.0151) construction
  line L146 (21.2954, -17.4638) -> (23.4263, -17.4638) construction
  line L147 (23.4263, -17.4638) -> (23.4263, -18.2657) construction
  line L148 (23.4263, -18.2657) -> (21.2954, -18.2657) construction
  line L149 (21.2954, -18.2657) -> (21.2954, -17.4638) construction
  line L150 (21.6556, 12.4414) -> (23.7866, 12.4414) construction
  line L151 (23.7866, 12.4414) -> (23.7866, 11.6394) construction
  line L152 (23.7866, 11.6394) -> (21.6556, 11.6394) construction
  line L153 (21.6556, 11.6394) -> (21.6556, 12.4414) construction
  line L154 (21.65, -9.3602) -> (21.65, -8.5582) construction
  line L155 (21.65, -8.5582) -> (23.781, -8.5582) construction
  line L156 (23.781, -8.5582) -> (23.781, -9.3602) construction
  line L157 (23.781, -9.3602) -> (21.65, -9.3602) construction
  line L158 (20.2031, -6.8543) -> (20.2031, -6.0524) construction
  line L159 (20.2031, -6.0524) -> (22.334, -6.0524) construction
  line L160 (22.334, -6.0524) -> (22.334, -6.8543) construction
  line L161 (22.334, -6.8543) -> (20.2031, -6.8543) construction
  line L162 (28.0868, -2.1973) -> (28.0868, -1.3954) construction
  line L163 (28.0868, -1.3954) -> (30.2178, -1.3954) construction
  line L164 (30.2178, -1.3954) -> (30.2178, -2.1973) construction
  line L165 (30.2178, -2.1973) -> (28.0868, -2.1973) construction
  line L166 (43.9941, -28.4266) -> (43.9941, -27.6247) construction
  line L167 (43.9941, -27.6247) -> (46.1251, -27.6247) construction
  line L168 (46.1251, -27.6247) -> (46.1251, -28.4266) construction
  line L169 (46.1251, -28.4266) -> (43.9941, -28.4266) construction
  line L170 (44.059, 27.912) -> (44.059, 28.714) construction
  line L171 (44.059, 28.714) -> (46.19, 28.714) construction
  line L172 (46.19, 28.714) -> (46.19, 27.912) construction
  line L173 (46.19, 27.912) -> (44.059, 27.912) construction
  line L174 (30.8118, -1.6727) -> (30.8118, -0.8708) construction
  line L175 (30.8118, -0.8708) -> (32.9427, -0.8708) construction
  line L176 (32.9427, -0.8708) -> (32.9427, -1.6727) construction
  line L177 (32.9427, -1.6727) -> (30.8118, -1.6727) construction
  line L178 (31.0967, 0.7575) -> (31.0967, 1.5594) construction
  line L179 (31.0967, 1.5594) -> (33.2276, 1.5594) construction
  line L180 (33.2276, 1.5594) -> (33.2276, 0.7575) construction
  line L181 (33.2276, 0.7575) -> (31.0967, 0.7575) construction
  line L182 (-45.9605, -28.4422) -> (-45.9605, -27.6403) construction
  line L183 (-45.9605, -27.6403) -> (-43.8296, -27.6403) construction
  line L184 (-43.8296, -27.6403) -> (-43.8296, -28.4422) construction
  line L185 (-43.8296, -28.4422) -> (-45.9605, -28.4422) construction
  line L186 (-46.2808, 27.6214) -> (-46.2808, 28.4233) construction
  line L187 (-46.2808, 28.4233) -> (-44.1498, 28.4233) construction
  line L188 (-44.1498, 28.4233) -> (-44.1498, 27.6214) construction
  line L189 (-44.1498, 27.6214) -> (-46.2808, 27.6214) construction
  line L190 (-24.3879, 21.6861) -> (-24.3879, 22.4881) construction
  line L191 (-24.3879, 22.4881) -> (-22.257, 22.4881) construction
  line L192 (-22.257, 22.4881) -> (-22.257, 21.6861) construction
  line L193 (-22.257, 21.6861) -> (-24.3879, 21.6861) construction
  line L194 (-24.302, -22.2794) -> (-24.302, -21.4774) construction
  line L195 (-24.302, -21.4774) -> (-22.1711, -21.4774) construction
  line L196 (-22.1711, -21.4774) -> (-22.1711, -22.2794) construction
  line L197 (-22.1711, -22.2794) -> (-24.302, -22.2794) construction
  spline S0 degree 2 poles (28.5646, -1.9776) (28.5646, -2.0294) (28.529, -2.1215) (28.4933, -2.1539) knots 0 0 0 1 2 2 2
  spline S1 degree 2 poles (28.4933, -2.1539) (28.4531, -2.1902) (28.3435, -2.2246) (28.2722, -2.2246) knots 0 0 0 1 2 2 2
  spline S2 degree 2 poles (28.2722, -2.2246) (28.2191, -2.2246) (28.1257, -2.2168) (28.0901, -2.209) knots 0 0 0 1 2 2 2
  line L198 (28.0901, -2.209) -> (28.0901, -2.0469)
  line L199 (28.0901, -2.0469) -> (28.1082, -2.0469)
  spline S3 degree 2 poles (28.1082, -2.0469) (28.1322, -2.0567) (28.1847, -2.0735) (28.2262, -2.0735) knots 0 0 0 1 2 2 2
  spline S4 degree 2 poles (28.2262, -2.0735) (28.2794, -2.0735) (28.3371, -2.0437) (28.3487, -2.0165) knots 0 0 0 1 2 2 2
  spline S5 degree 2 poles (28.3487, -2.0165) (28.361, -1.9899) (28.3636, -1.9212) (28.3636, -1.8784) knots 0 0 0 1 2 2 2
  line L200 (28.3636, -1.8784) -> (28.3636, -1.5575)
  line L201 (28.3636, -1.5575) -> (28.1808, -1.5575)
  line L202 (28.1808, -1.5575) -> (28.1808, -1.4123)
  line L203 (28.1808, -1.4123) -> (28.5646, -1.4123)
  line L204 (28.5646, -1.4123) -> (28.5646, -1.9776)
  spline S6 degree 2 poles (29.2862, -1.9698) (29.2862, -2.0288) (29.2427, -2.1254) (29.2006, -2.1591) knots 0 0 0 1 2 2 2
  spline S7 degree 2 poles (29.2006, -2.1591) (29.1584, -2.1928) (29.0437, -2.2291) (28.9614, -2.2291) knots 0 0 0 1 2 2 2
  spline S8 degree 2 poles (28.9614, -2.2291) (28.868, -2.2291) (28.7345, -2.198) (28.6923, -2.1785) knots 0 0 0 1 2 2 2
  line L205 (28.6923, -2.1785) -> (28.6923, -2.0048)
  line L206 (28.6923, -2.0048) -> (28.7118, -2.0048)
  spline S9 degree 2 poles (28.7118, -2.0048) (28.7559, -2.0327) (28.8745, -2.0742) (28.9238, -2.0742) knots 0 0 0 1 2 2 2
  spline S10 degree 2 poles (28.9238, -2.0742) (28.9529, -2.0742) (29.021, -2.0638) (29.0443, -2.0469) knots 0 0 0 1 2 2 2
  spline S11 degree 2 poles (29.0443, -2.0469) (29.0625, -2.0333) (29.0845, -1.9938) (29.0845, -1.9581) knots 0 0 0 1 2 2 2
  spline S12 degree 2 poles (29.0845, -1.9581) (29.0845, -1.9225) (29.0534, -1.8842) (29.0275, -1.8751) knots 0 0 0 1 2 2 2
  spline S13 degree 2 poles (29.0275, -1.8751) (29.0016, -1.8661) (28.9296, -1.8641) (28.9017, -1.8641) knots 0 0 0 1 2 2 2
  line L207 (28.9017, -1.8641) -> (28.8674, -1.8641)
  line L208 (28.8674, -1.8641) -> (28.8674, -1.7234)
  line L209 (28.8674, -1.7234) -> (28.8991, -1.7234)
  spline S14 degree 2 poles (28.8991, -1.7234) (28.9354, -1.7234) (28.997, -1.717) (29.0184, -1.7072) knots 0 0 0 1 2 2 2
  spline S15 degree 2 poles (29.0184, -1.7072) (29.0398, -1.6969) (29.0638, -1.6606) (29.0638, -1.6294) knots 0 0 0 1 2 2 2
  spline S16 degree 2 poles (29.0638, -1.6294) (29.0638, -1.6048) (29.0411, -1.5743) (29.0249, -1.5659) knots 0 0 0 1 2 2 2
  spline S17 degree 2 poles (29.0249, -1.5659) (29.0054, -1.5562) (28.9536, -1.5497) (28.9354, -1.5497) knots 0 0 0 1 2 2 2
  spline S18 degree 2 poles (28.9354, -1.5497) (28.9063, -1.5497) (28.8447, -1.5633) (28.8161, -1.5743) knots 0 0 0 1 2 2 2
  spline S19 degree 2 poles (28.8161, -1.5743) (28.7935, -1.5828) (28.7442, -1.61) (28.7325, -1.6171) knots 0 0 0 1 2 2 2
  line L210 (28.7325, -1.6171) -> (28.7157, -1.6171)
  line L211 (28.7157, -1.6171) -> (28.7157, -1.446)
  spline S20 degree 2 poles (28.7157, -1.446) (28.7572, -1.4285) (28.8972, -1.3954) (28.9704, -1.3954) knots 0 0 0 1 2 2 2
  spline S21 degree 2 poles (28.9704, -1.3954) (29.0418, -1.3954) (29.1468, -1.42) (29.1837, -1.444) knots 0 0 0 1 2 2 2
  spline S22 degree 2 poles (29.1837, -1.444) (29.2246, -1.4693) (29.2654, -1.5471) (29.2654, -1.5957) knots 0 0 0 1 2 2 2
  spline S23 degree 2 poles (29.2654, -1.5957) (29.2654, -1.6644) (29.1863, -1.7669) (29.1215, -1.7818) knots 0 0 0 1 2 2 2
  line L212 (29.1215, -1.7818) -> (29.1215, -1.7896)
  spline S24 degree 2 poles (29.1215, -1.7896) (29.15, -1.7935) (29.2045, -1.8142) (29.2304, -1.8375) knots 0 0 0 1 2 2 2
  spline S25 degree 2 poles (29.2304, -1.8375) (29.2544, -1.8583) (29.2862, -1.9244) (29.2862, -1.9698) knots 0 0 0 1 2 2 2
  line L213 (31.5696, -1.6708) -> (31.3687, -1.6708)
  line L214 (31.3687, -1.6708) -> (31.3687, -1.3162)
  line L215 (31.3687, -1.3162) -> (31.0957, -1.3162)
  line L216 (31.0957, -1.3162) -> (31.0957, -1.6708)
  line L217 (31.0957, -1.6708) -> (30.8947, -1.6708)
  line L218 (30.8947, -1.6708) -> (30.8947, -0.8708)
  line L219 (30.8947, -0.8708) -> (31.0957, -0.8708)
  line L220 (31.0957, -0.8708) -> (31.0957, -1.1638)
  line L221 (31.0957, -1.1638) -> (31.3687, -1.1638)
  line L222 (31.3687, -1.1638) -> (31.3687, -0.8708)
  line L223 (31.3687, -0.8708) -> (31.5696, -0.8708)
  line L224 (31.5696, -0.8708) -> (31.5696, -1.6708)
  spline S26 degree 2 poles (32.3035, -1.3998) (32.3035, -1.4627) (32.2607, -1.569) (32.2186, -1.6073) knots 0 0 0 1 2 2 2
  spline S27 degree 2 poles (32.2186, -1.6073) (32.1764, -1.6455) (32.061, -1.6876) (31.9768, -1.6876) knots 0 0 0 1 2 2 2
  spline S28 degree 2 poles (31.9768, -1.6876) (31.8873, -1.687) (31.7589, -1.6578) (31.7168, -1.639) knots 0 0 0 1 2 2 2
  line L225 (31.7168, -1.639) -> (31.7168, -1.4646)
  line L226 (31.7168, -1.4646) -> (31.7349, -1.4646)
  spline S29 degree 2 poles (31.7349, -1.4646) (31.7505, -1.4731) (31.7881, -1.4951) (31.8186, -1.5068) knots 0 0 0 1 2 2 2
  spline S30 degree 2 poles (31.8186, -1.5068) (31.8471, -1.5178) (31.9061, -1.5327) (31.9418, -1.5327) knots 0 0 0 1 2 2 2
  spline S31 degree 2 poles (31.9418, -1.5327) (31.9729, -1.5327) (32.0455, -1.5171) (32.0675, -1.4964) knots 0 0 0 1 2 2 2
  spline S32 degree 2 poles (32.0675, -1.4964) (32.0837, -1.4802) (32.1019, -1.4406) (32.1019, -1.4076) knots 0 0 0 1 2 2 2
  spline S33 degree 2 poles (32.1019, -1.4076) (32.1019, -1.3791) (32.0785, -1.3389) (32.0597, -1.3265) knots 0 0 0 1 2 2 2
  spline S34 degree 2 poles (32.0597, -1.3265) (32.0325, -1.3084) (31.9547, -1.298) (31.9268, -1.298) knots 0 0 0 1 2 2 2
  spline S35 degree 2 poles (31.9268, -1.298) (31.8828, -1.298) (31.7991, -1.3123) (31.7687, -1.3201) knots 0 0 0 1 2 2 2
  line L227 (31.7687, -1.3201) -> (31.7512, -1.3201)
  line L228 (31.7512, -1.3201) -> (31.7512, -0.8708)
  line L229 (31.7512, -0.8708) -> (32.2815, -0.8708)
  line L230 (32.2815, -0.8708) -> (32.2815, -1.0218)
  line L231 (32.2815, -1.0218) -> (31.9411, -1.0218)
  line L232 (31.9411, -1.0218) -> (31.9411, -1.1547)
  spline S36 degree 2 poles (31.9411, -1.1547) (31.9573, -1.1534) (32.002, -1.1521) (32.0144, -1.1521) knots 0 0 0 1 2 2 2
  spline S37 degree 2 poles (32.0144, -1.1521) (32.0721, -1.1521) (32.1693, -1.1755) (32.2076, -1.1995) knots 0 0 0 1 2 2 2
  spline S38 degree 2 poles (32.2076, -1.1995) (32.2529, -1.2293) (32.3035, -1.3285) (32.3035, -1.3998) knots 0 0 0 1 2 2 2
  line L233 (31.8545, 0.7445) -> (31.6535, 0.7445)
  line L234 (31.6535, 0.7445) -> (31.6535, 1.0991)
  line L235 (31.6535, 1.0991) -> (31.3806, 1.0991)
  line L236 (31.3806, 1.0991) -> (31.3806, 0.7445)
  line L237 (31.3806, 0.7445) -> (31.1796, 0.7445)
  line L238 (31.1796, 0.7445) -> (31.1796, 1.5445)
  line L239 (31.1796, 1.5445) -> (31.3806, 1.5445)
  line L240 (31.3806, 1.5445) -> (31.3806, 1.2515)
  line L241 (31.3806, 1.2515) -> (31.6535, 1.2515)
  line L242 (31.6535, 1.2515) -> (31.6535, 1.5445)
  line L243 (31.6535, 1.5445) -> (31.8545, 1.5445)
  line L244 (31.8545, 1.5445) -> (31.8545, 0.7445)
  spline S39 degree 2 poles (32.602, 1.0168) (32.602, 0.8904) (32.4419, 0.7277) (32.3018, 0.7277) knots 0 0 0 1 2 2 2
  spline S40 degree 2 poles (32.3018, 0.7277) (32.2318, 0.7277) (32.1223, 0.7679) (32.084, 0.8074) knots 0 0 0 1 2 2 2
  spline S41 degree 2 poles (32.084, 0.8074) (32.0386, 0.8534) (31.99, 0.9993) (31.99, 1.1011) knots 0 0 0 1 2 2 2
  spline S42 degree 2 poles (31.99, 1.1011) (31.99, 1.2061) (32.0354, 1.3695) (32.0866, 1.4324) knots 0 0 0 1 2 2 2
  spline S43 degree 2 poles (32.0866, 1.4324) (32.1352, 1.492) (32.2934, 1.5594) (32.4017, 1.5594) knots 0 0 0 1 2 2 2
  spline S44 degree 2 poles (32.4017, 1.5594) (32.4412, 1.5594) (32.5203, 1.5491) (32.5346, 1.5458) knots 0 0 0 1 2 2 2
  line L245 (32.5346, 1.5458) -> (32.5346, 1.3889)
  line L246 (32.5346, 1.3889) -> (32.5203, 1.3889)
  spline S45 degree 2 poles (32.5203, 1.3889) (32.5061, 1.3961) (32.4412, 1.4136) (32.3997, 1.4136) knots 0 0 0 1 2 2 2
  spline S46 degree 2 poles (32.3997, 1.4136) (32.3057, 1.4136) (32.2033, 1.3144) (32.191, 1.2223) knots 0 0 0 1 2 2 2
  spline S47 degree 2 poles (32.191, 1.2223) (32.2305, 1.2476) (32.3116, 1.2774) (32.3628, 1.2774) knots 0 0 0 1 2 2 2
  spline S48 degree 2 poles (32.3628, 1.2774) (32.4062, 1.2774) (32.4821, 1.2541) (32.5112, 1.232) knots 0 0 0 1 2 2 2
  spline S49 degree 2 poles (32.5112, 1.232) (32.5527, 1.2003) (32.602, 1.0972) (32.602, 1.0168) knots 0 0 0 1 2 2 2
  spline S50 degree 2 poles (32.368, 0.8962) (32.3835, 0.9157) (32.4004, 0.9611) (32.4004, 1.0071) knots 0 0 0 1 2 2 2
  spline S51 degree 2 poles (32.4004, 1.0071) (32.4004, 1.046) (32.3809, 1.0966) (32.3634, 1.1115) knots 0 0 0 1 2 2 2